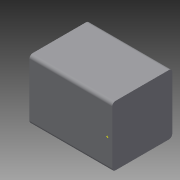
# Autodesk Inventor part: G723-280-4
Saved by Autodesk Inventor 2013 (Build 170138000, 138)
## iProperties
Created: 2012-11-28
Part Number: G723-280-4
Material: Generic
Document SubType Name: Modeling
Designer: istvan.burbank
Density: 1 g/cm^3
Mass: 258.816 g
Surface Area: 246.452 cm^2
Volume: 258.816 cm^3
Author: istvan.burbank
Autodesk Inventor part; units mm, degrees
ref_plane "YZ Plane" through (0, 0, 0) normal (1, 0, 0) x (0, 1, 0)
ref_plane "XZ Plane" through (0, 0, 0) normal (0, 1, 0) x (-1, 0, 0)
ref_plane "XY Plane" through (0, 0, 0) normal (0, 0, 1) x (1, 0, 0)
sketch "Sketch1" plane through (0, 0, 0) normal (1, 0, 0) x (0, 1, 0)
  line L0 (3.175, 0) -> (53.975, 0)
  line L1 (57.15, 3.175) -> (57.15, 53.975)
  line L2 (53.975, 57.15) -> (3.175, 57.15)
  line L3 (0, 53.975) -> (0, 3.175)
  arc A0 (3.175, 57.15) -> (0, 53.975) centre (3.175, 53.975) ccw
  arc A1 (57.15, 53.975) -> (53.975, 57.15) centre (53.975, 53.975) ccw
  arc A2 (53.975, 0) -> (57.15, 3.175) centre (53.975, 3.175) ccw
  arc A3 (0, 3.175) -> (3.175, 0) centre (3.175, 3.175) ccw
  point P0 (0, 0)
  point P1 (57.15, 57.15)
  point P2 (57.15, 0)
  point P3 (0, 57.15)
  dimension "d0" = 57.15
  dimension "d1" = 57.15
  dimension "d17" = 3.175
  constraints: 8 end point, 8 point on circle, 8 point on line, 8 tangent, 4 centre point, 3 equal radius, 2 parallel, 1 horizontal, 1 perpendicular
  measures "d0" distance of point (0, 57.15) point (57.15, 57.15)
  measures "d1" distance of point (57.15, 57.15) point (57.15, 0)
  measures "d17" radius of A0
extrude "Extrusion1" add sketch "Sketch1" along normal blind 78.74
sketch "Sketch2" plane through (0, 0, 0) normal (-1, 0, 0) x (0, 0, 1)
  line L0 (0, 53.975) -> (0, 3.175) projected
  line L1 (53.975, 57.15) -> (3.175, 57.15) projected
  circle A0 centre (28.575, 28.575) radius 19.05
  point P0 (0, 57.15)
  point P1 (0, 0)
  point P2 (57.15, 57.15)
  dimension "d4" = 38.1
  dimension "d18" = 28.575
  dimension "d19" = 28.575
  constraints: 1 centre point
  measures "d4" diameter of A0
  measures "d18" distance from line of L1 A0.centre
  measures "d19" distance from line of L0 A0.centre
extrude "Extrusion2" add sketch "Sketch2" along normal blind 1.524
sketch "Sketch3" plane through (-1.524, 28.575, 28.575) normal (-1, 0, 0) x (0, 0, 1)
  circle A0 centre (0, 0) radius 19.05 projected
  circle A1 centre (0, 0) radius 3.175
  point P0 (-28.575, -28.575)
  dimension "d10" = 6.35
  constraints: 1 centre point, 1 coincident
  measures "d10" diameter of A1
extrude "Extrusion3" add sketch "Sketch3" along normal blind 19.05 contours A1
sketch "Sketch4" plane through (-20.574, 28.575, 28.575) normal (-1, 0, 0) x (0, 0, 1)
  circle A0 centre (0, 0) radius 3.175 projected
  line L0 (-1.7227, 2.667) -> (1.7227, 2.667)
  line L1 (0, -3.175) -> (-5.2914, -3.175)
  point P0 (-28.575, -28.575)
  dimension "d13" = 5.842
  constraints: 4 end point, 3 point on circle, 1 horizontal, 1 parallel, 1 tangent
  measures "d13" distance between parallel lines of L0 L1
extrude "Extrusion4" cut sketch "Sketch4" against normal blind 14.986 contours L0 A0 picked at (-0.1211, 2.8294)
body "Solid1"
